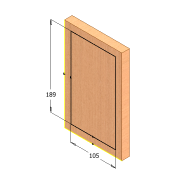
# Autodesk Inventor part: PRC-7-infoboard
Saved by Autodesk Inventor 2020 (Build 240168000, 168)
## iProperties
Created: 2021-06-23
Part Number: PRC-7-infoboard
Material: Generic
Document SubType Name: Modeling
Designer: Aidan Lee
Density: 1 g/cm^3
Appearance: Cherry - Natural Low Gloss
Author: Aidan Lee
Autodesk Inventor part; units mm, degrees
ref_plane "YZ Plane" through (0, 0, 0) normal (1, 0, 0) x (0, 1, 0)
ref_plane "XZ Plane" through (0, 0, 0) normal (0, 1, 0) x (-1, 0, 0)
ref_plane "XY Plane" through (0, 0, 0) normal (0, 0, 1) x (1, 0, 0)
sketch "Sketch1" plane through (0, 0, 0) normal (0, 0, 1) x (1, 0, 0)
  line L0 (0, 0) -> (135, 0)
  line L1 (135, 0) -> (135, 219)
  line L2 (135, 219) -> (0, 219)
  line L3 (0, 219) -> (0, 0)
  dimension "d1" = 219
  dimension "d2" = 135
  constraints: 8 end point, 2 parallel, 1 horizontal, 1 perpendicular
  measures "d1" distance of L2.end L0.start
  measures "d2" distance of L0.start L0.end
extrude "Extrusion1" add sketch "Sketch1" along normal blind 18
sketch "Sketch2" plane through (0, 0, 18) normal (0, 0, 1) x (1, 0, 0)
  line L0 (15, 204) -> (120, 204)
  line L1 (120, 204) -> (120, 15)
  line L2 (120, 15) -> (15, 15)
  line L3 (15, 15) -> (15, 204)
  line L4 (0, 219) -> (0, 0) projected
  line L5 (0, 0) -> (135, 0) projected
  point P0 (0, 109.5)
  point P1 (15, 109.5)
  point P2 (67.5, 15)
  point P3 (67.5, 0)
  dimension "d5" = 105
  dimension "d6" = 189
  constraints: 8 end point, 4 midpoint, 2 parallel, 1 horizontal, 1 horizontal alignment, 1 perpendicular, 1 vertical alignment
  measures "d5" distance of L1.end L2.end
  measures "d6" distance of L2.end L0.start
body "Solid1"
